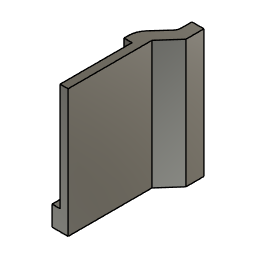
Banner Stand Hook Part  A v1 (Autodesk Fusion 360 design; units mm, degrees)
Autodesk Fusion 360 part; units mm, degrees
sketch "Sketch1" plane through (0, 0, 0) normal (0, 0, 1) x (1, 0, 0)
  line L0 (0, 0) -> (0, -4.5)
  line L1 (-16, -9) -> (18, -9) construction
  line L2 (0, -4.5) -> (-4, -9)
  line L3 (-4, -9) -> (-4, -30)
  line L4 (0, 0) -> (-3, 0)
  line L5 (-3, 0) -> (-3, -2.7268)
  line L6 (-4, -30) -> (-8, -30)
  line L7 (-8, -30) -> (-8, -10.933)
  line L8 (-3.5201, -4.0721) -> (-6.6997, -7.5697)
  arc A0 (-3.5201, -4.0721) -> (-3, -2.7268) centre (-5, -2.7268) ccw
  arc A1 (-6.6997, -7.5697) -> (-8, -10.933) centre (-3, -10.933) ccw
  point P0 (-3, -3.5)
  dimension "d1" = 4.5
  dimension "d2" = 4.5
  dimension "d3" = 21
  dimension "d4" = 3
  dimension "d5" = 3.5
  dimension "d6" = 4
  dimension "d7" = 2
  dimension "d8" = 5
  constraint coincident L0.start L4.start
  constraint vertical L0
  constraint horizontal L1
  constraint coincident L1 L2.end
  constraint perpendicular L1 L3
  constraint horizontal L4
  constraint perpendicular L4 L5
  constraint perpendicular L3 L6
  constraint perpendicular L1 L7
  constraint coincident P0 L5
  constraint coincident P0 L8
  constraint tangent L5 A0
  constraint tangent L8 A0
  constraint tangent L8 A1
  constraint tangent L7 A1
  measures "d1" distance of L0.start L0.end
  measures "d2" distance of L0.end L1
  measures "d3" distance of L2.end L3.end
  measures "d4" distance of L0.start L4.end
  measures "d5" distance of L4.end P0
  measures "d6" distance of L3.end L6.end
  measures "d7" radius of A0
  measures "d8" radius of A1
extrude "Extrude1" add sketch "Sketch1" along normal blind 32
sketch "Sketch2" plane through (-8, 0, 0) normal (-1, 0, 0) x (0, -1, 0)
  line L0 (10.933, 0) -> (30, 0)
  line L1 (30, 0) -> (30, 32)
  line L2 (30, 32) -> (10.933, 32)
  line L3 (10.933, 32) -> (10.933, 0)
  line L4 (30, 0) -> (15, 0)
  line L5 (15, 0) -> (15, 32)
  line L6 (15, 32) -> (30, 32)
  line L7 (30, 32) -> (30, 0)
  dimension "d11" = 15
  constraint horizontal L4
  constraint vertical L5
  constraint horizontal L6
  constraint vertical L7
  constraint coincident L2 L5.end
  constraint coincident L0.end L1.start
  measures "d11" distance of L0.end L4.end
extrude "Extrude2" add sketch "Sketch2" along normal blind 22 contours L0 L1 L2 L4 L5 L6 L7
extrude "Extrude3" cut 1 faces at (-30, -20, 21.3333) along direction (1, 0, 0) blind 2
extrude "Extrude4" add 1 faces at (-21.3333, -15, 10.6667) along direction (0, 1, 0) blind 4
extrude "Extrude5" cut 1 faces at (-21.3333, -11, 10.6667) along direction (0, -1, 0) blind 50
sketch "Sketch4" plane through (-8, 0, 0) normal (-1, 0, 0) x (0, -1, 0)
  line L0 (30, 0) -> (30, 32)
  line L1 (30, 32) -> (11, 32)
  line L2 (11, 32) -> (11, 0)
  line L3 (11, 0) -> (30, 0)
  line L4 (30, 32) -> (17, 32)
  line L5 (17, 32) -> (17, 5)
  line L6 (17, 5) -> (30, 5)
  line L7 (30, 5) -> (30, 32)
  dimension "d23" = 27
  constraint horizontal L4
  constraint vertical L5
  constraint horizontal L6
  constraint vertical L7
  constraint coincident L0.end L1.start
  measures "d23" distance of L0.end L6.end
extrude "Extrude6" cut sketch "Sketch4" against normal blind 2 contours L0 L1 L4 L5 L6 L7
extrude "Extrude7" cut 1 faces at (-7.3333, -17, 23) along direction (0, 1, 0) blind 5
